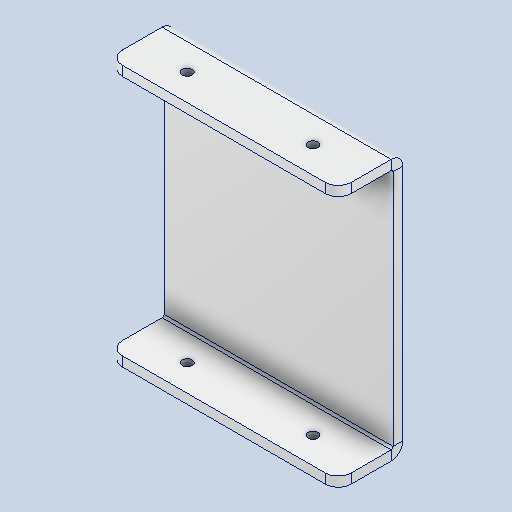
# Autodesk Inventor part: ㄷ_frame_3
Saved by Autodesk Inventor 2023 (Build 270158000, 158)
## iProperties
Created: 2022-10-29
Part Number: ㄷ_frame_3
Material: Aluminum 6061
Document SubType Name: Sheet Metal
Designer: chanh
Density: 2.7 g/cm^3
Sheet Metal Rule: Default_mm
Appearance: Aluminum - Flat
Flat Pattern Width: 3.55 cm
Flat Pattern Length: 5.50586 cm
Flat Pattern Area: 19.5458 cm^2
Sheet Metal Width: 35.500 mm
Sheet Metal Length: 55.059 mm
Sheet Metal Area: 1954.579 mm^2
품번: 21
Author: chanh
Autodesk Inventor part; units mm, degrees
note: some values were not read from the file. Chosen so that the rebuilt part matches the saved one: direction of "Hole1"; direction of "Hole2".
ref_plane "YZ Plane" through (0, 0, 0) normal (1, 0, 0) x (0, 1, 0)
ref_plane "XZ Plane" through (0, 0, 0) normal (0, 1, 0) x (-1, 0, 0)
ref_plane "XY Plane" through (0, 0, 0) normal (0, 0, 1) x (1, 0, 0)
sketch "Sketch1" plane through (0, 0, 0) normal (0, 0, 1) x (1, 0, 0)
  line L0 (-17.75, -20.25) -> (17.75, -20.25)
  line L1 (17.75, -20.25) -> (17.75, 20.25)
  line L2 (17.75, 20.25) -> (-17.75, 20.25)
  line L3 (-17.75, 20.25) -> (-17.75, -20.25)
  line L4 (-17.75, -20.25) -> (17.75, 20.25) construction
  line L5 (17.75, -20.25) -> (-17.75, 20.25) construction
  point P0 (0, 0)
  dimension "d0" = 35.5
  dimension "d1" = 40.5
  measures "d0" distance of L2.end L1.end
  measures "d1" distance of L1.end L0.end
extrude "Plate1" add sketch "Sketch1" along normal blind 1.5
sketch "Sketch2" plane through (-17.75, 18.75, 0) normal (0, 1, 0) x (-1, 0, 0)
  line L0 (-35.5, 0) -> (0, 0)
  line L1 (0, 0) -> (0, 10)
  line L2 (0, 10) -> (-35.5, 10)
  line L3 (-35.5, 10) -> (-35.5, 0)
  constraints: 6 end point, 1 horizontal, 1 perpendicular, 1 vertical
edge flange "Flange1" height 10 angle 90 thickness 1.5 bend radius 0.31 thickness toward (0, 1, 0) relief tear relief width 1.5 relief depth 0.75 corner gap 0.31 corner form 0 edges at (0, 20.25, 1.5) (0, -20.25, 1.5) wall of the first edge with corners at (17.75, 18.75, 0) (-17.75, 18.75, 0) (-17.75, 18.75, 10) (17.75, 18.75, 10)
bend "Bend1"
corner "Corner1"
sketch "Sketch3" plane through (-17.75, 20.25, 10) normal (0, 1, 0) x (1, 0, 0)
  line L0 (35.5, 8.19) -> (0, 8.19) projected
  line L1 (0, 0) -> (0, 8.19) projected
  line L2 (35.5, 0) -> (0, 0) projected
  line L3 (35.5, 8.19) -> (35.5, 0) projected
  point P0 (17.75, 10)
  point P1 (8, 4.095)
  point P2 (27.5, 4.095)
  point P3 (0, 4.095)
  point P4 (35.5, 4.095)
  dimension "d13" = 8
  dimension "d14" = 8
  constraints: 2 horizontal alignment, 2 midpoint
  measures "d13" distance from line of L1 point (8, 4.095)
  measures "d14" distance from line of point (27.5, 4.095) L3
hole "Hole1" at (-9.75, 20.25, 5.905) at (9.75, 20.25, 5.905) direction (0, -1, 0) diameter 1.567 depth 1.5 thread size "M2x0.4" class "6H" standard "ISO Metric profile"
sketch "Sketch4" plane through (-17.75, -20.25, 10) normal (0, -1, 0) x (1, 0, 0)
  circle A0 centre (27.5, -4.095) radius 0.7835 projected
  circle A1 centre (8, -4.095) radius 0.7835 projected
  point P0 (17.75, -10)
hole "Hole2" at (9.75, -20.25, 5.905) at (-9.75, -20.25, 5.905) direction (0, 1, 0) diameter 1.567 depth 1.5 thread size "M2x0.4" class "6H" standard "ISO Metric profile"
fillet "Corner Round1" radius 2 4 edges at (17.75, 19.5, 10) (-17.75, 19.5, 10) (17.75, -19.5, 10) (-17.75, -19.5, 10)
equation "\"d14\" = d13"
equation "\"d20\" = Thickness"
equation "\"d2\" = Thickness"
equation "\"d3\" = BendReliefWidth"
equation "\"d4\" = BendReliefDepth"
equation "\"d5\" = MinimumRemnant"
equation "\"d6\" = TransitionRadius"
equation "\"d9\" = BendRadius"
equation "\"d10\" = CornerReliefSize"
equation "\"d11\" = GapSize"
equation "\"d12\" = JacobiRadiusSize"
equation "\"BendReliefWidth\" = Thickness"
equation "\"BendReliefDepth\" = 0.5 * Thickness"
equation "\"CornerReliefSize\" = 4 * Thickness"
equation "\"MinimumRemnant\" = 2 * Thickness"
equation "\"TransitionRadius\" = BendRadius"
equation "\"JacobiRadiusSize\" = BendRadius"
equation "\"GapSize\" = Thickness"
equation "\"Thickness\" = 1.5"
equation "\"BendRadius\" = 0.31"
body "Solid1"
